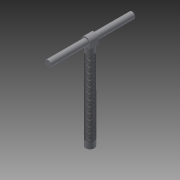
# Autodesk Inventor part: fuso
Saved by Autodesk Inventor 2015 (Build 190159000, 159)
## iProperties
Created: 2015-08-28
Part Number: fuso
Material: Generic
Document SubType Name: Modeling
Designer: EriveltonDell
Density: 1 g/cm^3
Appearance: Default
Author: EriveltonDell
Autodesk Inventor part; units mm, degrees
ref_plane "YZ Plane" through (0, 0, 0) normal (1, 0, 0) x (0, 1, 0)
ref_plane "XZ Plane" through (0, 0, 0) normal (0, 1, 0) x (-1, 0, 0)
ref_plane "XY Plane" through (0, 0, 0) normal (0, 0, 1) x (1, 0, 0)
sketch "Sketch1" plane through (0, 0, 0) normal (0, 1, 0) x (-1, 0, 0)
  circle A0 centre (0, 0) radius 35
  dimension "d0" = 70
  constraints: 1 centre point, 1 coincident
  measures "d0" diameter of A0
extrude "Extrusion1" add sketch "Sketch1" along normal blind 700
sketch "Sketch2" plane through (0, 700, 0) normal (0, 1, 0) x (1, 0, 0)
  line L0 (0, 0) -> (0, -35)
  line L1 (0, -35) -> (35, -35)
  line L2 (35, -35) -> (35, 35)
  line L3 (35, 35) -> (-35, 35)
  line L4 (-35, 35) -> (-35, -35)
  circle A0 centre (0, 0) radius 35 projected
  line L5 (-35, -35) -> (0, -35)
  dimension "d3" = 35
  dimension "d4" = 35
  dimension "d5" = 70
  dimension "d6" = 70
  dimension "d7" = 70
  constraints: 12 end point, 3 perpendicular, 1 point on line, 1 vertical
  measures "d3" distance of L0.start L0.end
  measures "d4" distance of L0.end L1.end
  measures "d5" distance of L1.end L2.end
  measures "d6" distance of L2.end L3.end
  measures "d7" distance of L3.end L4.end
extrude "Extrusion2" add sketch "Sketch2" along normal blind 70
sketch "Sketch3" plane through (-35, 700, 35) normal (0, 0, 1) x (1, 0, 0)
  circle A0 centre (35, 35) radius 25
  point P0 (35, -700)
  dimension "d10" = 50
  constraints: 1 centre point
  measures "d10" diameter of A0
extrude "Extrusion3" add sketch "Sketch3" along normal blind 300
sketch "Sketch4" plane through (35, 700, -35) normal (0, 0, -1) x (-1, 0, 0)
  line L0 (70, 70) -> (70, 35)
  line L1 (70, 0) -> (70, 70) projected
  line L2 (70, 35) -> (35, 35)
  circle A0 centre (35, 35) radius 25
  point P0 (35, -700)
  dimension "d13" = 35
  dimension "d14" = 35
  dimension "d15" = 50
  constraints: 4 end point, 1 centre point, 1 coincident, 1 midpoint, 1 perpendicular
  measures "d13" distance of L0.start L0.end
  measures "d14" distance of L0.end L2.end
  measures "d15" diameter of A0
extrude "Extrusion4" add sketch "Sketch4" along normal blind 300
fillet "Fillet1" radius 35 2 edges at (35, 770, 0) (-35, 770, 0)
thread "Thread1" size "M70x6" class "6g" standard "ANSI Metric M Profile" length 600 offset 50
body "Solid1"
